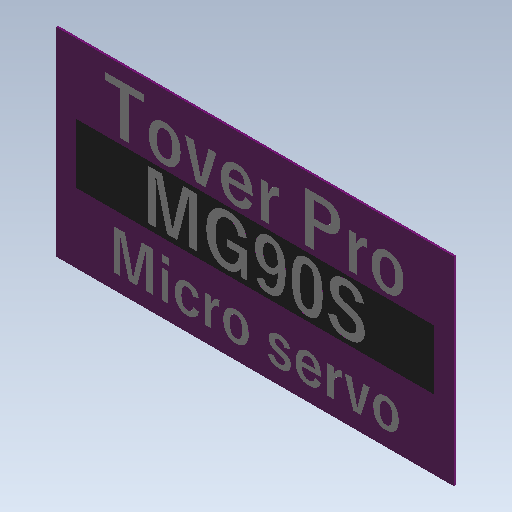
# Autodesk Inventor part: Этикетка
Saved by Autodesk Inventor 2020 (Build 240168000, 168)
## iProperties
Created: 2018-08-28
Part Number: Этикетка
Material: Пластик ПАЭК
Document SubType Name: Modeling
Designer: Shepelev
Density: 1.32 g/cm^3
Appearance: Гладкий - пурпурный
Author: Shepelev
Autodesk Inventor part; units mm, degrees
ref_plane "YZ Plane" through (0, 0, 0) normal (1, 0, 0) x (0, 1, 0)
ref_plane "XZ Plane" through (0, 0, 0) normal (0, 1, 0) x (-1, 0, 0)
ref_plane "XY Plane" through (0, 0, 0) normal (0, 0, 1) x (1, 0, 0)
sketch "Эскиз1" plane through (0, 0, 0) normal (0, 0, 1) x (1, 0, 0)
  line L0 (-10, -5) -> (10, -5)
  line L1 (10, -5) -> (10, 5)
  line L2 (10, 5) -> (-10, 5)
  line L3 (-10, 5) -> (-10, -5)
  line L4 (-10, -5) -> (10, 5) construction
  line L5 (10, -5) -> (-10, 5) construction
  point P0 (0, 0)
  dimension "d0" = 20
  dimension "d1" = 10
  constraints: 12 end point, 2 midpoint, 2 parallel, 1 horizontal, 1 perpendicular
  measures "d0" distance of L1.end L2.end
  measures "d1" distance of L2.end L0.start
extrude "Выдавливание1" add sketch "Эскиз1" along normal blind 0.1
sketch "Эскиз2" plane through (0, 0, 0.1) normal (0, 0, 1) x (1, 0, 0)
  line L0 (-9, -1.5) -> (9, -1.5)
  line L1 (9, -1.5) -> (9, 1.5)
  line L2 (9, 1.5) -> (-9, 1.5)
  line L3 (-9, 1.5) -> (-9, -1.5)
  line L4 (-9, -1.5) -> (9, 1.5) construction
  line L5 (9, -1.5) -> (-9, 1.5) construction
  point P0 (0, 0)
  dimension "d4" = 3
  dimension "d5" = 18
  constraints: 12 end point, 2 midpoint, 2 parallel, 1 horizontal, 1 perpendicular
  measures "d4" distance of L0.end L1.end
  measures "d5" distance of L1.end L2.end
emboss "Рельеф1" sketch "Эскиз2" operation add depth 0.0001 direction (0, 0, -1)
sketch "Эскиз3" plane through (0, 0, 0.1) normal (0, 0, 1) x (1, 0, 0)
  line L0 (-8, 4.5) -> (8, 4.5) construction
  line L1 (8, 4.5) -> (8, -4.5) construction
  line L2 (8, -4.5) -> (-8, -4.5) construction
  line L3 (-8, -4.5) -> (-8, 4.5) construction
  line L4 (-5.5976, 4.268) -> (-5.5976, 3.9175)
  line L5 (-5.5976, 3.9175) -> (-6.3412, 3.9175)
  line L6 (-6.3412, 3.9175) -> (-6.3412, 1.768)
  line L7 (-6.3412, 1.768) -> (-6.7808, 1.768)
  line L8 (-6.7808, 1.768) -> (-6.7808, 3.9175)
  line L9 (-6.7808, 3.9175) -> (-7.5182, 3.9175)
  line L10 (-7.5182, 3.9175) -> (-7.5182, 4.268)
  line L11 (-7.5182, 4.268) -> (-5.5976, 4.268)
  spline S0 degree 2 poles (-4.5401, 3.5772) (-4.1532, 3.5772) (-3.9344, 3.2976) knots 0 0 0 1 1 1
  spline S1 degree 2 poles (-3.9344, 3.2976) (-3.7399, 3.0504) (-3.7399, 2.6534) knots 0 0 0 1 1 1
  spline S2 degree 2 poles (-3.7399, 2.6534) (-3.7399, 2.1955) (-3.9891, 1.9402) knots 0 0 0 1 1 1
  spline S3 degree 2 poles (-3.9891, 1.9402) (-4.2018, 1.7214) (-4.5421, 1.7214) knots 0 0 0 1 1 1
  spline S4 degree 2 poles (-4.5421, 1.7214) (-4.9331, 1.7214) (-5.1499, 2.001) knots 0 0 0 1 1 1
  spline S5 degree 2 poles (-5.1499, 2.001) (-5.3424, 2.2462) (-5.3424, 2.6453) knots 0 0 0 1 1 1
  spline S6 degree 2 poles (-5.3424, 2.6453) (-5.3424, 3.1011) (-5.0912, 3.3584) knots 0 0 0 1 1 1
  spline S7 degree 2 poles (-5.0912, 3.3584) (-4.8764, 3.5772) (-4.5401, 3.5772) knots 0 0 0 1 1 1
  spline S8 degree 2 poles (-4.5401, 3.2855) (-4.9271, 3.2855) (-4.9271, 2.6513) knots 0 0 0 1 1 1
  spline S9 degree 2 poles (-4.9271, 2.6513) (-4.9271, 2.0152) (-4.5421, 2.0152) knots 0 0 0 1 1 1
  spline S10 degree 2 poles (-4.5421, 2.0152) (-4.1552, 2.0152) (-4.1552, 2.6513) knots 0 0 0 1 1 1
  spline S11 degree 2 poles (-4.1552, 2.6513) (-4.1552, 3.2855) (-4.5401, 3.2855) knots 0 0 0 1 1 1
  line L12 (-1.9348, 3.5367) -> (-2.4899, 1.768)
  line L13 (-2.4899, 1.768) -> (-2.97, 1.768)
  line L14 (-2.97, 1.768) -> (-3.519, 3.5367)
  line L15 (-3.519, 3.5367) -> (-3.0835, 3.5367)
  line L16 (-3.0835, 3.5367) -> (-2.8991, 2.7992)
  spline S12 degree 2 poles (-2.8991, 2.7992) (-2.8626, 2.6554) (-2.814, 2.4346) knots 0 0 0 1 1 1
  spline S13 degree 2 poles (-2.814, 2.4346) (-2.7573, 2.1955) (-2.737, 2.1104) knots 0 0 0 1 1 1
  line L17 (-2.737, 2.1104) -> (-2.7006, 2.1104)
  spline S14 degree 2 poles (-2.7006, 2.1104) (-2.6722, 2.2158) (-2.6074, 2.4791) knots 0 0 0 1 1 1
  spline S15 degree 2 poles (-2.6074, 2.4791) (-2.5567, 2.6817) (-2.5223, 2.8073) knots 0 0 0 1 1 1
  line L18 (-2.5223, 2.8073) -> (-2.3318, 3.5367)
  line L19 (-2.3318, 3.5367) -> (-1.9348, 3.5367)
  line L20 (-0.1216, 2.5642) -> (-1.3169, 2.5642)
  spline S16 degree 2 poles (-1.3169, 2.5642) (-1.3148, 2.2867) (-1.1872, 2.1388) knots 0 0 0 1 1 1
  spline S17 degree 2 poles (-1.1872, 2.1388) (-1.0737, 2.0051) (-0.8712, 2.0051) knots 0 0 0 1 1 1
  spline S18 degree 2 poles (-0.8712, 2.0051) (-0.5875, 2.0051) (-0.4984, 2.3414) knots 0 0 0 1 1 1
  line L21 (-0.4984, 2.3414) -> (-0.1297, 2.234)
  spline S19 degree 2 poles (-0.1297, 2.234) (-0.2978, 1.7214) (-0.8772, 1.7214) knots 0 0 0 1 1 1
  spline S20 degree 2 poles (-0.8772, 1.7214) (-1.3006, 1.7214) (-1.5194, 1.9949) knots 0 0 0 1 1 1
  spline S21 degree 2 poles (-1.5194, 1.9949) (-1.7139, 2.236) (-1.7139, 2.6412) knots 0 0 0 1 1 1
  spline S22 degree 2 poles (-1.7139, 2.6412) (-1.7139, 3.1011) (-1.4627, 3.3564) knots 0 0 0 1 1 1
  spline S23 degree 2 poles (-1.4627, 3.3564) (-1.2459, 3.5772) (-0.9117, 3.5772) knots 0 0 0 1 1 1
  spline S24 degree 2 poles (-0.9117, 3.5772) (-0.5369, 3.5772) (-0.3201, 3.3037) knots 0 0 0 1 1 1
  spline S25 degree 2 poles (-0.3201, 3.3037) (-0.1216, 3.0565) (-0.1216, 2.6473) knots 0 0 0 1 1 1
  line L22 (-0.1216, 2.6473) -> (-0.1216, 2.5642)
  spline S26 degree 2 poles (-0.5166, 2.8316) (-0.547, 3.2976) (-0.9056, 3.2976) knots 0 0 0 1 1 1
  spline S27 degree 2 poles (-0.9056, 3.2976) (-1.0981, 3.2976) (-1.2054, 3.1558) knots 0 0 0 1 1 1
  spline S28 degree 2 poles (-1.2054, 3.1558) (-1.2966, 3.0342) (-1.3108, 2.8316) knots 0 0 0 1 1 1
  line L23 (-1.3108, 2.8316) -> (-0.5166, 2.8316)
  line L24 (1.2156, 3.5772) -> (1.1892, 3.1963)
  spline S29 degree 2 poles (1.1892, 3.1963) (0.8509, 3.1963) (0.6868, 2.7466) knots 0 0 0 1 1 1
  line L25 (0.6868, 2.7466) -> (0.6868, 1.768)
  line L26 (0.6868, 1.768) -> (0.2877, 1.768)
  line L27 (0.2877, 1.768) -> (0.2877, 3.5367)
  line L28 (0.2877, 3.5367) -> (0.6686, 3.5367)
  line L29 (0.6686, 3.5367) -> (0.6686, 3.1031)
  spline S30 degree 2 poles (0.6686, 3.1031) (0.8408, 3.5772) (1.2156, 3.5772) knots 0 0 0 1 1 1
  line L30 (2.5101, 4.268) -> (3.3914, 4.268)
  spline S31 degree 2 poles (3.3914, 4.268) (4.2848, 4.268) (4.2848, 3.5529) knots 0 0 0 1 1 1
  spline S32 degree 2 poles (4.2848, 3.5529) (4.2848, 3.1801) (4.0194, 2.9876) knots 0 0 0 1 1 1
  spline S33 degree 2 poles (4.0194, 2.9876) (3.7804, 2.8175) (3.3651, 2.8175) knots 0 0 0 1 1 1
  line L31 (3.3651, 2.8175) -> (2.9437, 2.8175)
  line L32 (2.9437, 2.8175) -> (2.9437, 1.768)
  line L33 (2.9437, 1.768) -> (2.5101, 1.768)
  line L34 (2.5101, 1.768) -> (2.5101, 4.268)
  line L35 (2.9437, 3.9419) -> (2.9437, 3.1436)
  line L36 (2.9437, 3.1436) -> (3.3529, 3.1436)
  spline S34 degree 2 poles (3.3529, 3.1436) (3.8452, 3.1436) (3.8452, 3.5488) knots 0 0 0 1 1 1
  spline S35 degree 2 poles (3.8452, 3.5488) (3.8452, 3.9419) (3.3691, 3.9419) knots 0 0 0 1 1 1
  line L37 (3.3691, 3.9419) -> (2.9437, 3.9419)
  line L38 (5.6321, 3.5772) -> (5.6058, 3.1963)
  spline S36 degree 2 poles (5.6058, 3.1963) (5.2674, 3.1963) (5.1033, 2.7466) knots 0 0 0 1 1 1
  line L39 (5.1033, 2.7466) -> (5.1033, 1.768)
  line L40 (5.1033, 1.768) -> (4.7042, 1.768)
  line L41 (4.7042, 1.768) -> (4.7042, 3.5367)
  line L42 (4.7042, 3.5367) -> (5.0851, 3.5367)
  line L43 (5.0851, 3.5367) -> (5.0851, 3.1031)
  spline S37 degree 2 poles (5.0851, 3.1031) (5.2573, 3.5772) (5.6321, 3.5772) knots 0 0 0 1 1 1
  spline S38 degree 2 poles (6.6633, 3.5772) (7.0502, 3.5772) (7.269, 3.2976) knots 0 0 0 1 1 1
  spline S39 degree 2 poles (7.269, 3.2976) (7.4635, 3.0504) (7.4635, 2.6534) knots 0 0 0 1 1 1
  spline S40 degree 2 poles (7.4635, 2.6534) (7.4635, 2.1955) (7.2143, 1.9402) knots 0 0 0 1 1 1
  spline S41 degree 2 poles (7.2143, 1.9402) (7.0016, 1.7214) (6.6613, 1.7214) knots 0 0 0 1 1 1
  spline S42 degree 2 poles (6.6613, 1.7214) (6.2703, 1.7214) (6.0535, 2.001) knots 0 0 0 1 1 1
  spline S43 degree 2 poles (6.0535, 2.001) (5.861, 2.2462) (5.861, 2.6453) knots 0 0 0 1 1 1
  spline S44 degree 2 poles (5.861, 2.6453) (5.861, 3.1011) (6.1122, 3.3584) knots 0 0 0 1 1 1
  spline S45 degree 2 poles (6.1122, 3.3584) (6.327, 3.5772) (6.6633, 3.5772) knots 0 0 0 1 1 1
  spline S46 degree 2 poles (6.6633, 3.2855) (6.2763, 3.2855) (6.2763, 2.6513) knots 0 0 0 1 1 1
  spline S47 degree 2 poles (6.2763, 2.6513) (6.2763, 2.0152) (6.6613, 2.0152) knots 0 0 0 1 1 1
  spline S48 degree 2 poles (6.6613, 2.0152) (7.0482, 2.0152) (7.0482, 2.6513) knots 0 0 0 1 1 1
  spline S49 degree 2 poles (7.0482, 2.6513) (7.0482, 3.2855) (6.6633, 3.2855) knots 0 0 0 1 1 1
  line L44 (-2.9092, 1.268) -> (-2.9092, -1.232)
  line L45 (-2.9092, -1.232) -> (-3.3246, -1.232)
  line L46 (-3.3246, -1.232) -> (-3.3246, 0.0322)
  spline S50 degree 2 poles (-3.3246, 0.0322) (-3.3246, 0.3199) (-3.3165, 0.9135) knots 0 0 0 1 1 1
  line L47 (-3.3165, 0.9135) -> (-3.363, 0.9135)
  spline S51 degree 2 poles (-3.363, 0.9135) (-3.4846, 0.3705) (-3.5697, 0.0626) knots 0 0 0 1 1 1
  line L48 (-3.5697, 0.0626) -> (-3.908, -1.232)
  line L49 (-3.908, -1.232) -> (-4.4165, -1.232)
  line L50 (-4.4165, -1.232) -> (-4.7447, 0.0464)
  spline S52 degree 2 poles (-4.7447, 0.0464) (-4.7751, 0.1598) (-4.9575, 0.9135) knots 0 0 0 1 1 1
  line L51 (-4.9575, 0.9135) -> (-5.002, 0.9135)
  spline S53 degree 2 poles (-5.002, 0.9135) (-4.9939, 0.4799) (-4.9939, 0.0241) knots 0 0 0 1 1 1
  line L52 (-4.9939, 0.0241) -> (-4.9939, -1.232)
  line L53 (-4.9939, -1.232) -> (-5.3768, -1.232)
  line L54 (-5.3768, -1.232) -> (-5.3768, 1.268)
  line L55 (-5.3768, 1.268) -> (-4.6718, 1.268)
  line L56 (-4.6718, 1.268) -> (-4.3558, -0.0083)
  spline S54 degree 2 poles (-4.3558, -0.0083) (-4.2484, -0.4338) (-4.1754, -0.8329) knots 0 0 0 1 1 1
  line L57 (-4.1754, -0.8329) -> (-4.1288, -0.8329)
  spline S55 degree 2 poles (-4.1288, -0.8329) (-4.1025, -0.7275) (-4.0296, -0.4013) knots 0 0 0 1 1 1
  spline S56 degree 2 poles (-4.0296, -0.4013) (-3.9749, -0.1663) (-3.9364, -0.0144) knots 0 0 0 1 1 1
  line L58 (-3.9364, -0.0144) -> (-3.6163, 1.268)
  line L59 (-3.6163, 1.268) -> (-2.9092, 1.268)
  line L60 (-0.4092, 0.5792) -> (-0.8327, 0.4779)
  spline S57 degree 2 poles (-0.8327, 0.4779) (-0.9279, 0.9763) (-1.3513, 0.9763) knots 0 0 0 1 1 1
  spline S58 degree 2 poles (-1.3513, 0.9763) (-1.6653, 0.9763) (-1.8335, 0.7008) knots 0 0 0 1 1 1
  spline S59 degree 2 poles (-1.8335, 0.7008) (-1.9854, 0.4516) (-1.9854, 0.014) knots 0 0 0 1 1 1
  spline S60 degree 2 poles (-1.9854, 0.014) (-1.9854, -0.4824) (-1.7929, -0.7336) knots 0 0 0 1 1 1
  spline S61 degree 2 poles (-1.7929, -0.7336) (-1.6288, -0.9463) (-1.3574, -0.9463) knots 0 0 0 1 1 1
  spline S62 degree 2 poles (-1.3574, -0.9463) (-0.8651, -0.9463) (-0.7982, -0.2656) knots 0 0 0 1 1 1
  line L61 (-0.7982, -0.2656) -> (-1.3837, -0.2656)
  line L62 (-1.3837, -0.2656) -> (-1.3837, 0.0687)
  line L63 (-1.3837, 0.0687) -> (-0.393, 0.0687)
  line L64 (-0.393, 0.0687) -> (-0.393, -1.2482)
  line L65 (-0.393, -1.2482) -> (-0.6827, -1.2482)
  line L66 (-0.6827, -1.2482) -> (-0.7314, -0.8855)
  spline S63 degree 2 poles (-0.7314, -0.8855) (-0.8327, -1.0902) (-1.0251, -1.1935) knots 0 0 0 1 1 1
  spline S64 degree 2 poles (-1.0251, -1.1935) (-1.1912, -1.2806) (-1.4019, -1.2806) knots 0 0 0 1 1 1
  spline S65 degree 2 poles (-1.4019, -1.2806) (-1.9125, -1.2806) (-2.1941, -0.8997) knots 0 0 0 1 1 1
  spline S66 degree 2 poles (-2.1941, -0.8997) (-2.4473, -0.5594) (-2.4473, 0.012) knots 0 0 0 1 1 1
  spline S67 degree 2 poles (-2.4473, 0.012) (-2.4473, 0.6603) (-2.1029, 1.0128) knots 0 0 0 1 1 1
  spline S68 degree 2 poles (-2.1029, 1.0128) (-1.8132, 1.3106) (-1.3574, 1.3106) knots 0 0 0 1 1 1
  spline S69 degree 2 poles (-1.3574, 1.3106) (-0.9522, 1.3106) (-0.6969, 1.0837) knots 0 0 0 1 1 1
  spline S70 degree 2 poles (-0.6969, 1.0837) (-0.4862, 0.8953) (-0.4092, 0.5792) knots 0 0 0 1 1 1
  spline S71 degree 2 poles (0.4518, -0.7336) (0.5166, -0.9686) (0.7111, -0.9686) knots 0 0 0 1 1 1
  spline S72 degree 2 poles (0.7111, -0.9686) (0.938, -0.9686) (1.0454, -0.7437) knots 0 0 0 1 1 1
  spline S73 degree 2 poles (1.0454, -0.7437) (1.1467, -0.531) (1.1568, -0.0914) knots 0 0 0 1 1 1
  spline S74 degree 2 poles (1.1568, -0.0914) (1.0028, -0.3851) (0.6564, -0.3851) knots 0 0 0 1 1 1
  spline S75 degree 2 poles (0.6564, -0.3851) (0.3485, -0.3851) (0.1641, -0.142) knots 0 0 0 1 1 1
  spline S76 degree 2 poles (0.1641, -0.142) (0, 0.0727) (0, 0.409) knots 0 0 0 1 1 1
  spline S77 degree 2 poles (0, 0.409) (0, 0.8345) (0.2289, 1.0675) knots 0 0 0 1 1 1
  spline S78 degree 2 poles (0.2289, 1.0675) (0.4254, 1.268) (0.7415, 1.268) knots 0 0 0 1 1 1
  spline S79 degree 2 poles (0.7415, 1.268) (1.1487, 1.268) (1.3513, 0.9479) knots 0 0 0 1 1 1
  spline S80 degree 2 poles (1.3513, 0.9479) (1.5417, 0.6501) (1.5417, 0.0889) knots 0 0 0 1 1 1
  spline S81 degree 2 poles (1.5417, 0.0889) (1.5417, -0.6728) (1.2925, -1.0071) knots 0 0 0 1 1 1
  spline S82 degree 2 poles (1.2925, -1.0071) (1.0879, -1.2786) (0.703, -1.2786) knots 0 0 0 1 1 1
  spline S83 degree 2 poles (0.703, -1.2786) (0.2046, -1.2786) (0.0567, -0.8815) knots 0 0 0 1 1 1
  line L67 (0.0567, -0.8815) -> (0.4518, -0.7336)
  spline S84 degree 2 poles (1.1386, 0.2328) (1.1345, 0.9601) (0.7577, 0.9601) knots 0 0 0 1 1 1
  spline S85 degree 2 poles (0.7577, 0.9601) (0.4092, 0.9601) (0.4092, 0.4171) knots 0 0 0 1 1 1
  spline S86 degree 2 poles (0.4092, 0.4171) (0.4092, 0.17) (0.5146, 0.0383) knots 0 0 0 1 1 1
  spline S87 degree 2 poles (0.5146, 0.0383) (0.6037, -0.0752) (0.7476, -0.0752) knots 0 0 0 1 1 1
  spline S88 degree 2 poles (0.7476, -0.0752) (1.0028, -0.0752) (1.1386, 0.2328) knots 0 0 0 1 1 1
  spline S89 degree 2 poles (2.6297, 1.268) (3.0389, 1.268) (3.2273, 0.9358) knots 0 0 0 1 1 1
  spline S90 degree 2 poles (3.2273, 0.9358) (3.4015, 0.6258) (3.4015, 0.0038) knots 0 0 0 1 1 1
  spline S91 degree 2 poles (3.4015, 0.0038) (3.4015, -0.7073) (3.1746, -1.0192) knots 0 0 0 1 1 1
  spline S92 degree 2 poles (3.1746, -1.0192) (2.9842, -1.2786) (2.6216, -1.2786) knots 0 0 0 1 1 1
  spline S93 degree 2 poles (2.6216, -1.2786) (2.2083, -1.2786) (2.0219, -0.9402) knots 0 0 0 1 1 1
  spline S94 degree 2 poles (2.0219, -0.9402) (1.8517, -0.6282) (1.8517, -0.0022) knots 0 0 0 1 1 1
  spline S95 degree 2 poles (1.8517, -0.0022) (1.8517, 0.7068) (2.0806, 1.0148) knots 0 0 0 1 1 1
  spline S96 degree 2 poles (2.0806, 1.0148) (2.2711, 1.268) (2.6297, 1.268) knots 0 0 0 1 1 1
  spline S97 degree 2 poles (2.6297, 0.95) (2.421, 0.95) (2.342, 0.719) knots 0 0 0 1 1 1
  spline S98 degree 2 poles (2.342, 0.719) (2.267, 0.5022) (2.267, 0.0018) knots 0 0 0 1 1 1
  spline S99 degree 2 poles (2.267, 0.0018) (2.267, -0.5695) (2.3622, -0.7802) knots 0 0 0 1 1 1
  spline S100 degree 2 poles (2.3622, -0.7802) (2.4412, -0.9585) (2.6216, -0.9585) knots 0 0 0 1 1 1
  spline S101 degree 2 poles (2.6216, -0.9585) (2.8343, -0.9585) (2.9133, -0.7174) knots 0 0 0 1 1 1
  spline S102 degree 2 poles (2.9133, -0.7174) (2.9862, -0.4986) (2.9862, 0.0018) knots 0 0 0 1 1 1
  spline S103 degree 2 poles (2.9862, 0.0018) (2.9862, 0.5711) (2.893, 0.7757) knots 0 0 0 1 1 1
  spline S104 degree 2 poles (2.893, 0.7757) (2.814, 0.95) (2.6297, 0.95) knots 0 0 0 1 1 1
  line L68 (5.4801, 0.6886) -> (5.0567, 0.5731)
  spline S105 degree 2 poles (5.0567, 0.5731) (4.9595, 0.9824) (4.613, 0.9824) knots 0 0 0 1 1 1
  spline S106 degree 2 poles (4.613, 0.9824) (4.4024, 0.9824) (4.2889, 0.8831) knots 0 0 0 1 1 1
  spline S107 degree 2 poles (4.2889, 0.8831) (4.1957, 0.798) (4.1957, 0.6562) knots 0 0 0 1 1 1
  spline S108 degree 2 poles (4.1957, 0.6562) (4.1957, 0.4799) (4.3031, 0.3888) knots 0 0 0 1 1 1
  spline S109 degree 2 poles (4.3031, 0.3888) (4.4024, 0.3077) (4.6556, 0.2389) knots 0 0 0 1 1 1
  line L69 (4.6556, 0.2389) -> (4.7873, 0.1983)
  spline S110 degree 2 poles (4.7873, 0.1983) (5.2269, 0.0788) (5.389, -0.1137) knots 0 0 0 1 1 1
  spline S111 degree 2 poles (5.389, -0.1137) (5.5186, -0.2717) (5.5186, -0.5391) knots 0 0 0 1 1 1
  spline S112 degree 2 poles (5.5186, -0.5391) (5.5186, -0.9038) (5.2613, -1.1003) knots 0 0 0 1 1 1
  spline S113 degree 2 poles (5.2613, -1.1003) (5.0243, -1.2806) (4.6151, -1.2806) knots 0 0 0 1 1 1
  spline S114 degree 2 poles (4.6151, -1.2806) (4.22, -1.2806) (3.9749, -1.0983) knots 0 0 0 1 1 1
  spline S115 degree 2 poles (3.9749, -1.0983) (3.752, -0.9321) (3.671, -0.6323) knots 0 0 0 1 1 1
  line L70 (3.671, -0.6323) -> (4.0863, -0.5006)
  spline S116 degree 2 poles (4.0863, -0.5006) (4.139, -0.7316) (4.2889, -0.8491) knots 0 0 0 1 1 1
  spline S117 degree 2 poles (4.2889, -0.8491) (4.4206, -0.9524) (4.607, -0.9524) knots 0 0 0 1 1 1
  spline S118 degree 2 poles (4.607, -0.9524) (5.0851, -0.9524) (5.0851, -0.5958) knots 0 0 0 1 1 1
  spline S119 degree 2 poles (5.0851, -0.5958) (5.0851, -0.4155) (4.9797, -0.3284) knots 0 0 0 1 1 1
  spline S120 degree 2 poles (4.9797, -0.3284) (4.8764, -0.2413) (4.5968, -0.1623) knots 0 0 0 1 1 1
  line L71 (4.5968, -0.1623) -> (4.4672, -0.1238)
  spline S121 degree 2 poles (4.4672, -0.1238) (4.0498, -0.0002) (3.8938, 0.1923) knots 0 0 0 1 1 1
  spline S122 degree 2 poles (3.8938, 0.1923) (3.7642, 0.3523) (3.7642, 0.6278) knots 0 0 0 1 1 1
  spline S123 degree 2 poles (3.7642, 0.6278) (3.7642, 0.9439) (4.0093, 1.1343) knots 0 0 0 1 1 1
  spline S124 degree 2 poles (4.0093, 1.1343) (4.2342, 1.3106) (4.5989, 1.3106) knots 0 0 0 1 1 1
  spline S125 degree 2 poles (4.5989, 1.3106) (5.2816, 1.3106) (5.4801, 0.6886) knots 0 0 0 1 1 1
  line L72 (-5.1337, -2.2308) -> (-5.1337, -4.2308)
  line L73 (-5.1337, -4.2308) -> (-5.466, -4.2308)
  line L74 (-5.466, -4.2308) -> (-5.466, -3.2194)
  spline S126 degree 2 poles (-5.466, -3.2194) (-5.466, -2.9893) (-5.4595, -2.5144) knots 0 0 0 1 1 1
  line L75 (-5.4595, -2.5144) -> (-5.4968, -2.5144)
  spline S127 degree 2 poles (-5.4968, -2.5144) (-5.594, -2.9487) (-5.6621, -3.1951) knots 0 0 0 1 1 1
  line L76 (-5.6621, -3.1951) -> (-5.9327, -4.2308)
  line L77 (-5.9327, -4.2308) -> (-6.3395, -4.2308)
  line L78 (-6.3395, -4.2308) -> (-6.6021, -3.2081)
  spline S128 degree 2 poles (-6.6021, -3.2081) (-6.6264, -3.1173) (-6.7723, -2.5144) knots 0 0 0 1 1 1
  line L79 (-6.7723, -2.5144) -> (-6.8079, -2.5144)
  spline S129 degree 2 poles (-6.8079, -2.5144) (-6.8015, -2.8612) (-6.8015, -3.2259) knots 0 0 0 1 1 1
  line L80 (-6.8015, -3.2259) -> (-6.8015, -4.2308)
  line L81 (-6.8015, -4.2308) -> (-7.1078, -4.2308)
  line L82 (-7.1078, -4.2308) -> (-7.1078, -2.2308)
  line L83 (-7.1078, -2.2308) -> (-6.5438, -2.2308)
  line L84 (-6.5438, -2.2308) -> (-6.2909, -3.2518)
  spline S130 degree 2 poles (-6.2909, -3.2518) (-6.205, -3.5922) (-6.1467, -3.9115) knots 0 0 0 1 1 1
  line L85 (-6.1467, -3.9115) -> (-6.1094, -3.9115)
  spline S131 degree 2 poles (-6.1094, -3.9115) (-6.0883, -3.8272) (-6.03, -3.5662) knots 0 0 0 1 1 1
  spline S132 degree 2 poles (-6.03, -3.5662) (-5.9862, -3.3782) (-5.9554, -3.2567) knots 0 0 0 1 1 1
  line L86 (-5.9554, -3.2567) -> (-5.6994, -2.2308)
  line L87 (-5.6994, -2.2308) -> (-5.1337, -2.2308)
  line L88 (-4.3606, -2.8158) -> (-4.3606, -4.2308)
  line L89 (-4.3606, -4.2308) -> (-4.6864, -4.2308)
  line L90 (-4.6864, -4.2308) -> (-4.6864, -2.8158)
  line L91 (-4.6864, -2.8158) -> (-4.3606, -2.8158)
  line L92 (-4.3476, -2.2308) -> (-4.3476, -2.563)
  line L93 (-4.3476, -2.563) -> (-4.6977, -2.563)
  line L94 (-4.6977, -2.563) -> (-4.6977, -2.2308)
  line L95 (-4.6977, -2.2308) -> (-4.3476, -2.2308)
  line L96 (-2.816, -3.2356) -> (-3.1305, -3.3069)
  spline S133 degree 2 poles (-3.1305, -3.3069) (-3.1759, -3.0201) (-3.3817, -3.0201) knots 0 0 0 1 1 1
  spline S134 degree 2 poles (-3.3817, -3.0201) (-3.6994, -3.0201) (-3.6994, -3.5241) knots 0 0 0 1 1 1
  spline S135 degree 2 poles (-3.6994, -3.5241) (-3.6994, -4.0314) (-3.3817, -4.0314) knots 0 0 0 1 1 1
  spline S136 degree 2 poles (-3.3817, -4.0314) (-3.158, -4.0314) (-3.111, -3.7332) knots 0 0 0 1 1 1
  line L97 (-3.111, -3.7332) -> (-2.8096, -3.8158)
  spline S137 degree 2 poles (-2.8096, -3.8158) (-2.8647, -4.0509) (-3.0316, -4.1675) knots 0 0 0 1 1 1
  spline S138 degree 2 poles (-3.0316, -4.1675) (-3.1759, -4.268) (-3.3898, -4.268) knots 0 0 0 1 1 1
  spline S139 degree 2 poles (-3.3898, -4.268) (-3.7123, -4.268) (-3.8825, -4.046) knots 0 0 0 1 1 1
  spline S140 degree 2 poles (-3.8825, -4.046) (-4.0316, -3.8515) (-4.0316, -3.529) knots 0 0 0 1 1 1
  spline S141 degree 2 poles (-4.0316, -3.529) (-4.0316, -3.1594) (-3.8355, -2.9585) knots 0 0 0 1 1 1
  spline S142 degree 2 poles (-3.8355, -2.9585) (-3.6653, -2.7834) (-3.3898, -2.7834) knots 0 0 0 1 1 1
  spline S143 degree 2 poles (-3.3898, -2.7834) (-3.1451, -2.7834) (-2.9927, -2.9163) knots 0 0 0 1 1 1
  spline S144 degree 2 poles (-2.9927, -2.9163) (-2.8598, -3.033) (-2.816, -3.2356) knots 0 0 0 1 1 1
  line L98 (-1.7804, -2.7834) -> (-1.8015, -3.0881)
  spline S145 degree 2 poles (-1.8015, -3.0881) (-2.0721, -3.0881) (-2.2034, -3.4479) knots 0 0 0 1 1 1
  line L99 (-2.2034, -3.4479) -> (-2.2034, -4.2308)
  line L100 (-2.2034, -4.2308) -> (-2.5227, -4.2308)
  line L101 (-2.5227, -4.2308) -> (-2.5227, -2.8158)
  line L102 (-2.5227, -2.8158) -> (-2.218, -2.8158)
  line L103 (-2.218, -2.8158) -> (-2.218, -3.1627)
  spline S146 degree 2 poles (-2.218, -3.1627) (-2.0802, -2.7834) (-1.7804, -2.7834) knots 0 0 0 1 1 1
  spline S147 degree 2 poles (-0.9554, -2.7834) (-0.6459, -2.7834) (-0.4708, -3.0071) knots 0 0 0 1 1 1
  spline S148 degree 2 poles (-0.4708, -3.0071) (-0.3152, -3.2048) (-0.3152, -3.5225) knots 0 0 0 1 1 1
  spline S149 degree 2 poles (-0.3152, -3.5225) (-0.3152, -3.8888) (-0.5146, -4.093) knots 0 0 0 1 1 1
  spline S150 degree 2 poles (-0.5146, -4.093) (-0.6848, -4.268) (-0.9571, -4.268) knots 0 0 0 1 1 1
  spline S151 degree 2 poles (-0.9571, -4.268) (-1.2699, -4.268) (-1.4433, -4.0444) knots 0 0 0 1 1 1
  spline S152 degree 2 poles (-1.4433, -4.0444) (-1.5972, -3.8483) (-1.5972, -3.529) knots 0 0 0 1 1 1
  spline S153 degree 2 poles (-1.5972, -3.529) (-1.5972, -3.1643) (-1.3963, -2.9585) knots 0 0 0 1 1 1
  spline S154 degree 2 poles (-1.3963, -2.9585) (-1.2245, -2.7834) (-0.9554, -2.7834) knots 0 0 0 1 1 1
  spline S155 degree 2 poles (-0.9554, -3.0168) (-1.265, -3.0168) (-1.265, -3.5241) knots 0 0 0 1 1 1
  spline S156 degree 2 poles (-1.265, -3.5241) (-1.265, -4.033) (-0.9571, -4.033) knots 0 0 0 1 1 1
  spline S157 degree 2 poles (-0.9571, -4.033) (-0.6475, -4.033) (-0.6475, -3.5241) knots 0 0 0 1 1 1
  spline S158 degree 2 poles (-0.6475, -3.5241) (-0.6475, -3.0168) (-0.9554, -3.0168) knots 0 0 0 1 1 1
  line L104 (1.7739, -3.1449) -> (1.466, -3.234)
  spline S159 degree 2 poles (1.466, -3.234) (1.4141, -3.0055) (1.2147, -3.0055) knots 0 0 0 1 1 1
  spline S160 degree 2 poles (1.2147, -3.0055) (1.1062, -3.0055) (1.0446, -3.0557) knots 0 0 0 1 1 1
  spline S161 degree 2 poles (1.0446, -3.0557) (0.9927, -3.0962) (0.9927, -3.1578) knots 0 0 0 1 1 1
  spline S162 degree 2 poles (0.9927, -3.1578) (0.9927, -3.247) (1.0494, -3.2923) knots 0 0 0 1 1 1
  spline S163 degree 2 poles (1.0494, -3.2923) (1.1029, -3.3329) (1.2455, -3.3701) knots 0 0 0 1 1 1
  line L105 (1.2455, -3.3701) -> (1.3639, -3.4009)
  spline S164 degree 2 poles (1.3639, -3.4009) (1.6199, -3.469) (1.7172, -3.576) knots 0 0 0 1 1 1
  spline S165 degree 2 poles (1.7172, -3.576) (1.8031, -3.6716) (1.8031, -3.8321) knots 0 0 0 1 1 1
  spline S166 degree 2 poles (1.8031, -3.8321) (1.8031, -4.0444) (1.641, -4.1594) knots 0 0 0 1 1 1
  spline S167 degree 2 poles (1.641, -4.1594) (1.4903, -4.268) (1.2293, -4.268) knots 0 0 0 1 1 1
  spline S168 degree 2 poles (1.2293, -4.268) (0.7674, -4.268) (0.6394, -3.9131) knots 0 0 0 1 1 1
  line L106 (0.6394, -3.9131) -> (0.9408, -3.8077)
  spline S169 degree 2 poles (0.9408, -3.8077) (1.0089, -4.046) (1.2374, -4.046) knots 0 0 0 1 1 1
  spline S170 degree 2 poles (1.2374, -4.046) (1.4951, -4.046) (1.4951, -3.8628) knots 0 0 0 1 1 1
  spline S171 degree 2 poles (1.4951, -3.8628) (1.4951, -3.7721) (1.4352, -3.7316) knots 0 0 0 1 1 1
  spline S172 degree 2 poles (1.4352, -3.7316) (1.3833, -3.6975) (1.2229, -3.6505) knots 0 0 0 1 1 1
  line L107 (1.2229, -3.6505) -> (1.1045, -3.6181)
  spline S173 degree 2 poles (1.1045, -3.6181) (0.8582, -3.5517) (0.7674, -3.4463) knots 0 0 0 1 1 1
  spline S174 degree 2 poles (0.7674, -3.4463) (0.688, -3.3523) (0.688, -3.187) knots 0 0 0 1 1 1
  spline S175 degree 2 poles (0.688, -3.187) (0.688, -2.9957) (0.8436, -2.8855) knots 0 0 0 1 1 1
  spline S176 degree 2 poles (0.8436, -2.8855) (0.9862, -2.7834) (1.2196, -2.7834) knots 0 0 0 1 1 1
  spline S177 degree 2 poles (1.2196, -2.7834) (1.6524, -2.7834) (1.7739, -3.1449) knots 0 0 0 1 1 1
  line L108 (3.3152, -3.5938) -> (2.359, -3.5938)
  spline S178 degree 2 poles (2.359, -3.5938) (2.3606, -3.8158) (2.4627, -3.9342) knots 0 0 0 1 1 1
  spline S179 degree 2 poles (2.4627, -3.9342) (2.5535, -4.0411) (2.7156, -4.0411) knots 0 0 0 1 1 1
  spline S180 degree 2 poles (2.7156, -4.0411) (2.9425, -4.0411) (3.0138, -3.7721) knots 0 0 0 1 1 1
  line L109 (3.0138, -3.7721) -> (3.3088, -3.858)
  spline S181 degree 2 poles (3.3088, -3.858) (3.1742, -4.268) (2.7107, -4.268) knots 0 0 0 1 1 1
  spline S182 degree 2 poles (2.7107, -4.268) (2.372, -4.268) (2.1969, -4.0492) knots 0 0 0 1 1 1
  spline S183 degree 2 poles (2.1969, -4.0492) (2.0413, -3.8564) (2.0413, -3.5322) knots 0 0 0 1 1 1
  spline S184 degree 2 poles (2.0413, -3.5322) (2.0413, -3.1643) (2.2423, -2.9601) knots 0 0 0 1 1 1
  spline S185 degree 2 poles (2.2423, -2.9601) (2.4157, -2.7834) (2.6831, -2.7834) knots 0 0 0 1 1 1
  spline S186 degree 2 poles (2.6831, -2.7834) (2.983, -2.7834) (3.1564, -3.0022) knots 0 0 0 1 1 1
  spline S187 degree 2 poles (3.1564, -3.0022) (3.3152, -3.2) (3.3152, -3.5274) knots 0 0 0 1 1 1
  line L110 (3.3152, -3.5274) -> (3.3152, -3.5938)
  spline S188 degree 2 poles (2.9992, -3.3799) (2.9749, -3.0071) (2.688, -3.0071) knots 0 0 0 1 1 1
  spline S189 degree 2 poles (2.688, -3.0071) (2.534, -3.0071) (2.4481, -3.1205) knots 0 0 0 1 1 1
  spline S190 degree 2 poles (2.4481, -3.1205) (2.3752, -3.2178) (2.3639, -3.3799) knots 0 0 0 1 1 1
  line L111 (2.3639, -3.3799) -> (2.9992, -3.3799)
  line L112 (4.3849, -2.7834) -> (4.3639, -3.0881)
  spline S191 degree 2 poles (4.3639, -3.0881) (4.0932, -3.0881) (3.9619, -3.4479) knots 0 0 0 1 1 1
  line L113 (3.9619, -3.4479) -> (3.9619, -4.2308)
  line L114 (3.9619, -4.2308) -> (3.6426, -4.2308)
  line L115 (3.6426, -4.2308) -> (3.6426, -2.8158)
  line L116 (3.6426, -2.8158) -> (3.9473, -2.8158)
  line L117 (3.9473, -2.8158) -> (3.9473, -3.1627)
  spline S192 degree 2 poles (3.9473, -3.1627) (4.0851, -2.7834) (4.3849, -2.7834) knots 0 0 0 1 1 1
  line L118 (5.7658, -2.8158) -> (5.3217, -4.2308)
  line L119 (5.3217, -4.2308) -> (4.9376, -4.2308)
  line L120 (4.9376, -4.2308) -> (4.4984, -2.8158)
  line L121 (4.4984, -2.8158) -> (4.8468, -2.8158)
  line L122 (4.8468, -2.8158) -> (4.9943, -3.4058)
  spline S193 degree 2 poles (4.9943, -3.4058) (5.0235, -3.5209) (5.0624, -3.6975) knots 0 0 0 1 1 1
  spline S194 degree 2 poles (5.0624, -3.6975) (5.1078, -3.8888) (5.124, -3.9568) knots 0 0 0 1 1 1
  line L123 (5.124, -3.9568) -> (5.1532, -3.9568)
  spline S195 degree 2 poles (5.1532, -3.9568) (5.1759, -3.8726) (5.2277, -3.6619) knots 0 0 0 1 1 1
  spline S196 degree 2 poles (5.2277, -3.6619) (5.2682, -3.4998) (5.2958, -3.3993) knots 0 0 0 1 1 1
  line L124 (5.2958, -3.3993) -> (5.4481, -2.8158)
  line L125 (5.4481, -2.8158) -> (5.7658, -2.8158)
  spline S197 degree 2 poles (6.5843, -2.7834) (6.8938, -2.7834) (7.0689, -3.0071) knots 0 0 0 1 1 1
  spline S198 degree 2 poles (7.0689, -3.0071) (7.2245, -3.2048) (7.2245, -3.5225) knots 0 0 0 1 1 1
  spline S199 degree 2 poles (7.2245, -3.5225) (7.2245, -3.8888) (7.0251, -4.093) knots 0 0 0 1 1 1
  spline S200 degree 2 poles (7.0251, -4.093) (6.8549, -4.268) (6.5827, -4.268) knots 0 0 0 1 1 1
  spline S201 degree 2 poles (6.5827, -4.268) (6.2699, -4.268) (6.0964, -4.0444) knots 0 0 0 1 1 1
  spline S202 degree 2 poles (6.0964, -4.0444) (5.9425, -3.8483) (5.9425, -3.529) knots 0 0 0 1 1 1
  spline S203 degree 2 poles (5.9425, -3.529) (5.9425, -3.1643) (6.1434, -2.9585) knots 0 0 0 1 1 1
  spline S204 degree 2 poles (6.1434, -2.9585) (6.3152, -2.7834) (6.5843, -2.7834) knots 0 0 0 1 1 1
  spline S205 degree 2 poles (6.5843, -3.0168) (6.2747, -3.0168) (6.2747, -3.5241) knots 0 0 0 1 1 1
  spline S206 degree 2 poles (6.2747, -3.5241) (6.2747, -4.033) (6.5827, -4.033) knots 0 0 0 1 1 1
  spline S207 degree 2 poles (6.5827, -4.033) (6.8922, -4.033) (6.8922, -3.5241) knots 0 0 0 1 1 1
  spline S208 degree 2 poles (6.8922, -3.5241) (6.8922, -3.0168) (6.5843, -3.0168) knots 0 0 0 1 1 1
  point P0 (0, 0)
  point P1 (8, 0)
  point P2 (0, 4.5)
  dimension "d8" = 16
  dimension "d9" = 9
  constraints: 2 midpoint, 1 horizontal alignment, 1 vertical alignment, 2 other
  measures "d8" distance of L0.start L0.end
  measures "d9" distance of L0.end L1.end
emboss "Рельеф2" sketch "Эскиз3" operation cut depth 0.0002 direction (0, 0, -1)
